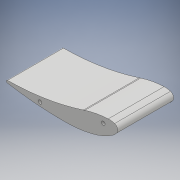
# Autodesk Inventor part: mainflap for side R
Saved by Autodesk Inventor 2018.3 (Build 223284000, 284)
## iProperties
Created: 2018-06-13
Part Number: mainflap for side R
Material: 一般
Document SubType Name: Modeling
Designer: ku_sk
Density: 1 g/cm^3
Appearance: 既定
Author: ku_sk
Autodesk Inventor part; units mm, degrees
ref_plane "YZ Plane" through (0, 0, 0) normal (1, 0, 0) x (0, 1, 0)
ref_plane "XZ Plane" through (0, 0, 0) normal (0, 1, 0) x (-1, 0, 0)
ref_plane "XY Plane" through (0, 0, 0) normal (0, 0, 1) x (1, 0, 0)
sketch "スケッチ2" plane through (0, 0, 0) normal (0, 1, 0) x (-1, 0, 0)
  arc A0 (186.0286, -63.1802) -> (352.6649, -47.4935) centre (165.9229, 1043.3137) ccw projected
  arc A1 (138.8299, -62.6406) -> (186.0286, -63.1802) centre (171.5405, 734.1521) ccw projected
  arc A2 (52.1426, -47.2314) -> (138.8299, -62.6406) centre (152.2575, 264.4411) ccw projected
  arc A3 (2.1008, -22.6524) -> (52.1426, -47.2314) centre (110.8425, 135.5101) ccw projected
  arc A4 (-12.1054, -8.8578) -> (2.1008, -22.6524) centre (35.5695, 26.0271) ccw projected
  arc A5 (-4.5779, 14.2844) -> (-12.1054, -8.8578) centre (0, 0) ccw projected
  arc A6 (16.7232, 17.0724) -> (-4.5779, 14.2844) centre (13.7336, -42.8531) ccw projected
  arc A7 (94.7165, 2.6851) -> (16.7232, 17.0724) centre (1.7751, -282.555) ccw projected
  arc A8 (94.7165, 2.6851) -> (99.4705, 1.147) centre (466.4821, 1143.6454) ccw projected
  arc A9 (99.4705, 1.147) -> (352.0248, -39.551) centre (359.437, 810.4167) ccw projected
  arc A10 (352.6649, -47.4935) -> (352.0248, -39.551) centre (351.99, -43.5508) ccw projected
  circle A11 centre (33.0346, -3.4541) radius 6 projected
  circle A12 centre (243.4846, -47.452) radius 6 projected
  point P0 (0, 0)
extrude "押し出し2" add sketch "スケッチ2" along normal mid plane 186
